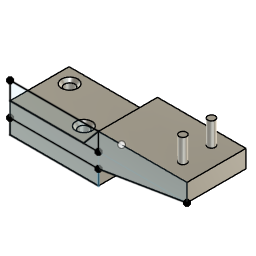
Halterung Türsensor Filamentschrank (Autodesk Fusion 360 design; units mm, degrees)
Autodesk Fusion 360 part; units mm, degrees
sketch "Skizze1" plane through (0, 0, 0) normal (0, 0, 1) x (1, 0, 0)
  line L0 (0, 0) -> (60, 0)
  line L1 (60, 0) -> (60, 20)
  line L2 (60, 20) -> (0, 20)
  line L3 (0, 20) -> (0, 0)
  circle A0 centre (53.2, 5.4) radius 1.275
  circle A1 centre (53.2, 15.1) radius 1.275
  line L4 (0, 20) -> (30, 20)
  line L5 (30, 20) -> (30, 0)
  line L6 (30, 0) -> (0, 0)
  line L7 (0, 0) -> (0, 20)
  dimension "d1" = 60
  dimension "d2" = 20
  dimension "d3" = 2.55
  dimension "d4" = 2.55
  dimension "d5" = 5.4
  dimension "d6" = 6.8
  dimension "d7" = 4.9
  dimension "d8" = 6.8
  constraint horizontal L0
  constraint vertical L1
  constraint horizontal L2
  constraint vertical L3
  constraint coincident L0.start L3.end
  constraint horizontal L4
  constraint vertical L5
  constraint horizontal L6
  constraint vertical L7
  constraint midpoint L0 L5.end
  measures "d1" distance of L0.start L0.end
  measures "d2" distance of L0.start L2.end
  measures "d3" diameter of A0
  measures "d4" diameter of A1
  measures "d5" distance of L0 A0.centre
  measures "d6" distance of L1 A0.centre
  measures "d7" distance of L2 A1.centre
  measures "d8" distance of L1 A1.centre
extrude "Extrusion1" add sketch "Skizze1" along normal blind 6
extrude "Extrusion2" add sketch "Skizze1" along normal blind 14 contours A0 | A1
extrude "Extrusion3" add sketch "Skizze1" against normal blind 5 contours L0 L2 L3 L4 L5 L6 L7
sketch "Skizze2" plane through (0, 0, 0) normal (0, -1, 0) x (1, 0, 0)
  line L0 (30, 0) -> (60, 0)
  line L1 (60, 0) -> (60, 6)
  line L2 (60, 6) -> (0, 6)
  line L3 (0, 6) -> (0, -5)
  line L4 (0, -5) -> (30, -5)
  line L5 (30, -5) -> (30, 0)
  line L6 (30, -5) -> (60, 0)
  line L7 (0, 6) -> (30, 6)
  line L8 (30, 6) -> (30, 0)
  line L9 (30, 0) -> (0, 0)
  line L10 (0, 0) -> (0, 6)
  line L11 (30, 6) -> (24.9654, 0)
  line L12 (30, 6) -> (37.8324, 6) construction
  line L13 (0, -5) -> (30, -5)
  line L14 (30, -5) -> (30, -10)
  line L15 (30, -10) -> (0, -10)
  line L16 (0, -10) -> (0, -5)
  dimension "d41" = 130
  dimension "d44" = 5
  constraint coincident L4.end L5.start
  constraint coincident L0.end L1.start
  constraint horizontal L7
  constraint vertical L8
  constraint horizontal L9
  constraint vertical L10
  constraint coincident L0.start L5.end
  constraint coincident L2.end L3.start
  constraint horizontal L12
  constraint coincident L9 L11.end
  constraint horizontal L13
  constraint vertical L14
  constraint horizontal L15
  constraint vertical L16
  constraint coincident L3.end L4.start
  measures "d41" angle of L11 L12
  measures "d44" distance of L3.end L15.end
extrude "Extrusion6" add sketch "Skizze2" against normal blind 20 contours L0 L5 L6
extrude "Extrusion7" cut sketch "Skizze2" against normal blind 20 contours L2 L3 L7 L9 L10 L11
extrude "Extrusion8" add sketch "Skizze2" against normal blind 20 contours L4 L13 L14 L15 L16
hole "Bohrung5" at (5.0685, 15.1186, 0) direction (0, 0, -1) diameter 3.5 depth 10 tip angle 180 countersink diameter 5.5 countersink angle 90
hole "Bohrung6" at (19.9516, 5.0738, 0) direction (0, 0, -1) diameter 3.5 depth 10 tip angle 180 countersink diameter 5.5 countersink angle 90
equation "d6 = 5.7 mm + 1.1 mm"
equation "d8 = 5.7 mm + 1.1 mm"
